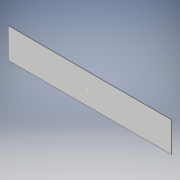
# Autodesk Inventor part: Faceplate
Saved by Autodesk Inventor 2017 (Build 210142000, 142)
## iProperties
Created: 2017-03-30
Part Number: Faceplate
Material: Generic
Document SubType Name: Modeling
Designer: plumbj
Density: 1 g/cm^3
Appearance: Default
Author: plumbj
Autodesk Inventor part; units mm, degrees
ref_plane "YZ Plane" through (0, 0, 0) normal (1, 0, 0) x (0, 1, 0)
ref_plane "XZ Plane" through (0, 0, 0) normal (0, 1, 0) x (-1, 0, 0)
ref_plane "XY Plane" through (0, 0, 0) normal (0, 0, 1) x (1, 0, 0)
sketch "Sketch1" plane through (0, 0, 0) normal (0, 0, 1) x (1, 0, 0)
  line L0 (-233.8021, -42.1254) -> (248.7979, -42.1254)
  line L1 (248.7979, -42.1254) -> (248.7979, 46.7746)
  line L2 (248.7979, 46.7746) -> (-233.8021, 46.7746)
  line L3 (-233.8021, 46.7746) -> (-233.8021, -42.1254)
  point P0 (0, 0)
  dimension "d0" = 482.6
  dimension "d1" = 88.9
  constraints: 8 end point, 2 parallel, 1 horizontal, 1 perpendicular
  measures "d0" distance of L2.end L1.end
  measures "d1" distance of L1.end L0.end
extrude "Extrusion1" add sketch "Sketch1" along normal blind 1.1113
sketch "Sketch2" plane through (0, 0, 1.1113) normal (0, 0, 1) x (1, 0, 0)
  point P0 (0, 0)
body "Solid1"
